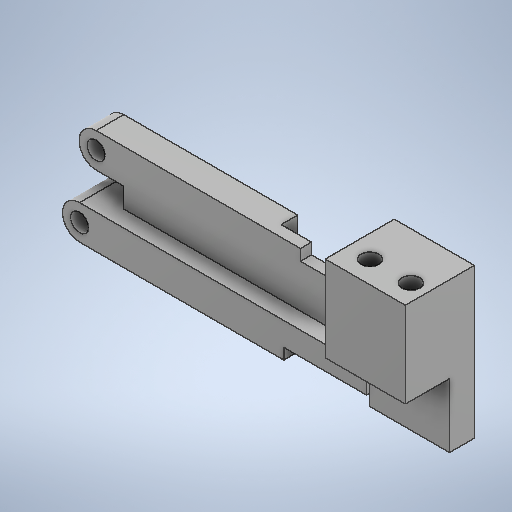
# Autodesk Inventor part: link_arm_5
Saved by Autodesk Inventor 2025 (Build 290162000, 162)
## iProperties
Created: 2025-09-16
Part Number: link_arm_5
Material: 一般
Document SubType Name: Modeling
Designer: sooo1
Density: 1 g/cm^3
Appearance: 滑らか - 標準の灰色
Author: sooo1
Autodesk Inventor part; units mm, degrees
ref_plane "YZ Plane" through (0, 0, 0) normal (1, 0, 0) x (0, 1, 0)
ref_plane "XZ Plane" through (0, 0, 0) normal (0, 1, 0) x (-1, 0, 0)
sketch "スケッチ1" plane through (0, 0, 0) normal (0, 0, 1) x (1, 0, 0)
  line L0 (-3, 8) -> (3, 8)
  line L1 (3, 8) -> (3, -8)
  line L2 (3, -8) -> (-3, -8)
  line L3 (-3, -8) -> (-3, 8)
  line L4 (-3, 8) -> (3, -8) construction
  line L5 (3, 8) -> (-3, -8) construction
  line L6 (0, 8) -> (0, -8) construction
  circle A0 centre (0, 4.9) radius 1.635
  circle A1 centre (0, -4.9) radius 1.635
  line L7 (0, 4.9) -> (0, -4.9)
  line L8 (-3, 0) -> (3, 0)
  circle A2 centre (0, 4.9) radius 3.1
  circle A3 centre (0, -4.9) radius 3.1
  line L9 (3, 8) -> (52, 8)
  line L10 (52, 8) -> (52, -8)
  line L11 (52, -8) -> (3, -8)
  line L12 (0, 1.8) -> (52, 1.8)
  line L13 (0, -1.8) -> (52, -1.8)
  line L14 (5, 8) -> (5, -8)
  point P0 (0, 0)
  point P1 (0, 0)
  point P2 (3, 1.8)
  point P3 (3, -1.8)
  dimension "d0" = 3.27
  dimension "d1" = 16
  dimension "d2" = 9.8
  dimension "d3" = 6
  dimension "d11" = 2
  dimension "d12" = 47
  constraints: 30 end point, 8 midpoint, 8 point on line, 4 centre point, 4 perpendicular, 4 point on circle, 3 parallel, 2 coincident, 2 horizontal, 2 tangent, 1 collinear, 1 equal radius, 1 vertical
  measures "d0" diameter of A0
  measures "d1" distance of L2.end L0.start
  measures "d2" distance of L7.end L7.start
  measures "d3" distance of L0.start L0.end
  measures "d11" distance between parallel lines of L1 L14
  measures "d12" distance between parallel lines of L14 L10
extrude "押し出し1" add sketch "スケッチ1" along normal blind 8 contours A3 L1 L3 | L3 A3 | A3 L1
ref_plane "作業平面1" through (0, 0, 5) normal (0, 0, -1) x (-1, 0, 0)
extrude "押し出し2" add sketch "スケッチ1" against normal blind 5 from surface at 5 contours A2 L1 L3 | L3 A2 | A2 L1
extrude "押し出し3" add sketch "スケッチ1" along normal up to surface (5 mm away) contours L9 L10 L12 L14 | L12 L10 L13 L14 | L13 L10 L11 L14
extrude "押し出し4" add sketch "スケッチ1" against normal up to surface (5 mm away) from surface at 5 contours L0 L1 A2 | L9 L14 L12 L1 A2 | L9 L10 L12 L14 | L1 L12 A2
extrude "押し出し5" add sketch "スケッチ1" along normal up to surface (8 mm away) contours L14 L11 L1 A3 L13 | L13 L10 L11 L14 | L13 L1 A3 | A3 L1 L2
sketch "スケッチ2" plane through (0, 0, 0) normal (0, 1, 0) x (-1, 0, 0)
  line L0 (-52, 0) -> (-52, 5) construction
  line L1 (-52, 23) -> (-66.5, 23)
  line L2 (-66.5, 23) -> (-66.5, 0)
  line L3 (-66.5, 0) -> (-52, 0)
  line L4 (-52, 0) -> (-52, 23)
  line L5 (-66.5, 11.5) -> (-52, 11.5) construction
  line L6 (-52, 17) -> (-66.5, 17)
  line L7 (-66.5, 17) -> (-66.5, 6)
  line L8 (-66.5, 6) -> (-52, 6)
  line L9 (-52, 6) -> (-52, 17)
  line L10 (-52, 17) -> (-66.5, 6) construction
  line L11 (-66.5, 17) -> (-52, 6) construction
  circle A0 centre (-56.1, 11.5) radius 1.635
  circle A1 centre (-63.5, 11.5) radius 1.635
  line L12 (-52, 15) -> (-66.5, 15) construction
  line L13 (-52, 0) -> (-5, 0) construction
  line L14 (-52, 0) -> (-52, 5) construction
  line L15 (0, 8) -> (-52, 8) construction
  line L16 (-52, 7.5) -> (-66.5, 7.5)
  line L17 (-53.1, 6) -> (-53.1, 17)
  line L18 (-59.25, 0) -> (-59.25, 23) construction
  line L19 (-52, 15.5) -> (-66.5, 15.5)
  line L20 (-65.4, 6) -> (-65.4, 17)
  line L21 (-53.1, 7.5) -> (-53.1, 15.5)
  point P0 (-59.25, 11.5)
  point P1 (-66.5, 17)
  point P2 (-65.4, 15.5)
  point P3 (-65.4, 7.5)
  point P4 (-66.5, 15.5)
  point P5 (-66.5, 7.5)
  point P6 (-52, 7.5)
  point P7 (-52, 15.5)
  dimension "d24" = 11
  dimension "d25" = 3.27
  dimension "d26" = 4.1
  dimension "d27" = 11.5
  dimension "d32" = 3.5
  dimension "d33" = 14.5
  dimension "d36" = 3.5
  dimension "d37" = 3
  dimension "d38" = 4
  constraints: 38 end point, 13 point on line, 9 midpoint, 4 collinear, 4 symmetric about line, 2 centre point, 2 horizontal, 2 perpendicular, 1 equal radius, 1 vertical
  measures "d24" distance of L6.end L7.end
  measures "d25" diameter of A0
  measures "d26" distance from line of L9 A0.centre
  measures "d27" distance from line of L9 A1.centre
  measures "d32" distance between parallel lines of L5 L12
  measures "d33" distance of L1.start L1.end
  measures "d36" distance between parallel lines of L5 L15
  measures "d37" distance from line of L17 A0.centre
  measures "d38" distance between parallel lines of L5 L16
extrude "押し出し7" add sketch "スケッチ2" along normal blind 30 from surface at -8
extrude "押し出し8" cut sketch "スケッチ2" against normal blind 12.5 from surface at 22 contours L4 L6 L2 L1 | L4 L19 L17 L6 | L6 L20 L19 L2 | L4 L16 L17 L19 | L17 L19 L20 L6 | L19 L20 L16 L2 | L4 L8 L17 L16 | L17 L16 L20 L19 | L16 L20 L8 L2 | L4 L3 L2 L8 | L17 L8 L20 L16 | A0 | A1
extrude "押し出し10" cut sketch "スケッチ2" along normal blind 11.6 from surface at -8 contours L4 L6 L2 L1 | L4 L19 L17 L6 | L6 L20 L19 L2 | L4 L16 L17 L19 | L17 L19 L20 L6 | L19 L20 L16 L2 | L17 L16 L20 L19
sketch "スケッチ4" plane through (0, 0, 0) normal (0, 0, -1) x (-1, 0, 0)
  circle A0 centre (0, 4.9) radius 1.635 projected
  circle A1 centre (0, -4.9) radius 1.635 projected
  line L0 (-52, 8) -> (-52, 9.5) projected
  line L1 (-52, 9.5) -> (-66.5, 9.5) projected
  line L2 (-66.5, -8) -> (-66.5, 9.5) projected
  line L3 (0, -8) -> (-66.5, -8) projected
  arc A2 (0, -8) -> (0, -1.8) centre (0, -4.9) ccw projected
  line L4 (-5, -1.8) -> (0, -1.8) projected
  line L5 (-5, 1.8) -> (-5, -1.8) projected
  line L6 (0, 1.8) -> (-5, 1.8) projected
  arc A3 (0, 1.8) -> (0, 8) centre (0, 4.9) ccw projected
  line L7 (-52, 8) -> (0, 8) projected
  line L8 (-52, 8) -> (-66.5, 8)
  line L9 (0, 0) -> (-66.5, 0) construction
  line L10 (-66.5, 8) -> (-31.5, 8)
  line L11 (-31.5, 8) -> (-31.5, -15)
  line L12 (-31.5, -15) -> (-66.5, -15)
  line L13 (-66.5, -15) -> (-66.5, 8)
  line L14 (-52, 8) -> (-37, 8)
  line L15 (-37, 8) -> (-37, 6)
  line L16 (-37, 6) -> (-52, 6)
  line L17 (-52, 6) -> (-52, 8)
  line L18 (-37, -8) -> (-37, -6)
  line L19 (-37, -6) -> (-52, -6)
  line L20 (-52, -6) -> (-52, -8)
  point P0 (-31.5, 8)
  point P1 (-37, 8)
  point P2 (-52, -8)
  point P3 (-37, -8)
  dimension "d41" = 35
  dimension "d42" = 23
  dimension "d43" = 15
  dimension "d44" = 2
  constraints: 26 end point, 4 parallel, 4 perpendicular, 4 symmetric about line, 2 horizontal, 2 point on line
  measures "d41" distance of L11.end L12.end
  measures "d42" distance of L12.end L8.end
  measures "d43" distance of L15.end L16.end
  measures "d44" distance between parallel lines of L7 L16
extrude "押し出し11" cut sketch "スケッチ4" against normal blind 3 contours L8 L2 L1 L0 | L17 L16 L15 L7 L11 L3 L18 L19 L20 L2 L8 | L7 L15 L16 L17 | L3 L11 L12 L13 | L20 L19 L18 L3
extrude "押し出し12" cut sketch "スケッチ4" against normal up to surface (8 mm away) contours L7 L15 L16 L17 | L20 L19 L18 L3
sketch "スケッチ5" plane through (52, 9.5, 23) normal (0, 1, 0) x (1, 0, 0)
  circle A0 centre (11.5, 11.5) radius 1.635 projected
  circle A1 centre (4.1, 11.5) radius 1.635 projected
  line L0 (14.5, 20) -> (0, 20) projected
  line L1 (0, 0) -> (0, 20) projected
  line L2 (14.5, 0) -> (0, 0) projected
  line L3 (14.5, 20) -> (14.5, 0) projected
  point P0 (-52, 23)
extrude "押し出し13" add sketch "スケッチ5" along normal blind 9.6
extrude "押し出し14" cut sketch "スケッチ2" along normal through all contours L4 L6 L2 L1 | L4 L19 L17 L6 | L6 L20 L19 L2 | L17 L19 L20 L6
